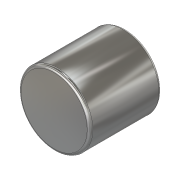
# Autodesk Inventor part: D44-N52
Saved by Autodesk Inventor 2019 (Build 230136000, 136)
## iProperties
Created: 2023-10-12
Part Number: D44-N52
Material: Nickel-Copper Alloy 400
Document SubType Name: Modeling
Designer: prich
Mass: 1.77092 g
Surface Area: 1.85608 cm^2
Volume: 0.200557 cm^3
Density: 8.83 g/cm^3
Appearance: Chrome - Polished
Author: prich
Autodesk Inventor part; units mm, degrees
ref_plane "YZ Plane" through (0, 0, 0) normal (1, 0, 0) x (0, 1, 0)
ref_plane "XZ Plane" through (0, 0, 0) normal (0, 1, 0) x (-1, 0, 0)
ref_plane "XY Plane" through (0, 0, 0) normal (0, 0, 1) x (1, 0, 0)
sketch "Sketch1" plane through (0, 0, 0) normal (0, 0, 1) x (1, 0, 0)
  circle A0 centre (0, 0) radius 3.175
  dimension "d0" = 6.35
  constraints: 1 centre point, 1 coincident
  measures "d0" diameter of A0
extrude "Extrusion1" add sketch "Sketch1" along normal blind 6.35
fillet "Fillet1" radius 0.254 2 edges at (-3.175, 0, 6.35) (-3.175, 0, 0)
body "Solid1"
